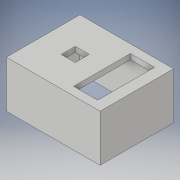
# Autodesk Inventor part: test_camAndultra
Saved by Autodesk Inventor 2018 (Build 220112000, 112)
## iProperties
Created: 2020-03-27
Part Number: test_camAndultra
Material: Generic
Document SubType Name: Modeling
Designer: natha
Density: 1 g/cm^3
Appearance: Default
Author: natha
Autodesk Inventor part; units mm, degrees
ref_plane "YZ Plane" through (0, 0, 0) normal (1, 0, 0) x (0, 1, 0)
ref_plane "XZ Plane" through (0, 0, 0) normal (0, 1, 0) x (-1, 0, 0)
ref_plane "XY Plane" through (0, 0, 0) normal (0, 0, 1) x (1, 0, 0)
sketch "Sketch1" plane through (0, 0, 0) normal (0, 1, 0) x (-1, 0, 0)
  line L0 (0, 0) -> (70, 0)
  line L1 (70, 0) -> (70, -55)
  line L2 (70, -55) -> (0, -55)
  line L3 (0, -55) -> (0, 0)
  line L4 (51.25, -32.75) -> (40.75, -32.75)
  line L5 (40.75, -32.75) -> (40.75, -22.25)
  line L6 (40.75, -22.25) -> (51.25, -22.25)
  line L7 (51.25, -22.25) -> (51.25, -32.75)
  line L8 (26, -48.75) -> (8, -48.75)
  line L9 (8, -48.75) -> (8, -6.25)
  line L10 (8, -6.25) -> (26, -6.25)
  line L11 (26, -6.25) -> (26, -48.75)
  dimension "d0" = 70
  dimension "d1" = 55
  dimension "d2" = 10.5
  dimension "d3" = 10.5
  dimension "d4" = 18
  dimension "d5" = 42.5
  dimension "d6" = 6.25
  dimension "d7" = 22.25
  dimension "d8" = 8
  dimension "d9" = 18.75
  constraints: 24 end point, 6 parallel, 3 horizontal, 3 perpendicular
  measures "d0" distance of L1.end L2.end
  measures "d1" distance of L0.end L1.end
  measures "d2" distance of L5.end L6.end
  measures "d3" distance of L4.end L5.end
  measures "d4" distance of L9.end L10.end
  measures "d5" distance of L8.end L9.end
  measures "d6" distance between parallel lines of L2 L8
  measures "d7" distance between parallel lines of L2 L4
  measures "d8" distance between parallel lines of L3 L9
  measures "d9" distance between parallel lines of L1 L7
extrude "Extrusion1" add sketch "Sketch1" along normal blind 4
sketch "Sketch2" plane through (0, 0, 0) normal (0, -1, 0) x (1, 0, 0)
  line L0 (0, 0) -> (0, -55) projected
  line L1 (-70, 0) -> (0, 0) projected
  line L2 (0, -55) -> (-70, -55)
  line L3 (-70, -55) -> (-70, 0)
  line L4 (-70, 0) -> (0, 0)
  line L5 (0, 0) -> (0, -55)
  line L6 (-3, -52) -> (-67, -52)
  line L7 (-67, -52) -> (-67, -3)
  line L8 (-67, -3) -> (-3, -3)
  line L9 (-3, -3) -> (-3, -52)
  line L10 (-29.5, -43.75) -> (-62.25, -43.75)
  line L11 (-62.25, -43.75) -> (-62.25, -11.25)
  line L12 (-62.25, -11.25) -> (-29.5, -11.25)
  line L13 (-40.75, -32.75) -> (-51.25, -32.75) projected
  line L14 (-51.25, -22.25) -> (-40.75, -22.25) projected
  line L15 (-51.25, -32.75) -> (-51.25, -22.25) projected
  line L16 (-40.75, -22.25) -> (-40.75, -32.75) projected
  line L17 (-29.5, -45.75) -> (-64.25, -45.75)
  line L18 (-64.25, -45.75) -> (-64.25, -9.25)
  line L19 (-64.25, -9.25) -> (-29.5, -9.25)
  line L20 (-29.5, -45.75) -> (-29.5, -43.75)
  line L21 (-29.5, -11.25) -> (-29.5, -9.25)
  dimension "d14" = 3
  dimension "d15" = 3
  dimension "d16" = 3
  dimension "d17" = 3
  dimension "d18" = 32.75
  dimension "d19" = 11
  dimension "d20" = 11
  dimension "d21" = 11
  dimension "d23" = 2
  dimension "d24" = 2
  dimension "d25" = 2
  constraints: 32 end point, 8 parallel, 4 horizontal, 4 perpendicular
  measures "d14" distance between parallel lines of L2 L6
  measures "d15" distance between parallel lines of L0 L9
  measures "d16" distance between parallel lines of L1 L8
  measures "d17" distance between parallel lines of L3 L7
  measures "d18" distance of L11.end L12.end
  measures "d19" distance between parallel lines of L10 L13
  measures "d20" distance between parallel lines of L14 L12
  measures "d21" distance between parallel lines of L11 L15
  measures "d23" distance between parallel lines of L17 L10
  measures "d24" distance between parallel lines of L18 L11
  measures "d25" distance between parallel lines of L12 L19
extrude "Extrusion2" add sketch "Sketch2" along normal blind 3 contours L20 L17 L18 L19 L21 L12 L11 L10
sketch "Sketch3" plane through (0, 0, 0) normal (0, -1, 0) x (1, 0, 0)
  line L0 (0, -55) -> (0, 0) projected
  line L1 (0, -55) -> (-70, -55)
  line L2 (-70, -55) -> (-70, 0)
  line L3 (-70, 0) -> (0, 0)
  line L4 (0, 0) -> (0, -55)
  line L5 (-3, -52) -> (-67, -52)
  line L6 (-67, -52) -> (-67, -3)
  line L7 (-67, -3) -> (-3, -3)
  line L8 (-3, -3) -> (-3, -52)
  dimension "d28" = 3
  dimension "d29" = 3
  dimension "d30" = 3
  dimension "d31" = 3
  constraints: 16 end point, 4 parallel, 2 horizontal, 2 perpendicular
  measures "d28" distance between parallel lines of L8 L0
  measures "d29" distance between parallel lines of L2 L6
  measures "d30" distance between parallel lines of L1 L5
  measures "d31" distance between parallel lines of L3 L7
extrude "Extrusion3" add sketch "Sketch3" along normal blind 31
body "Solid1"
